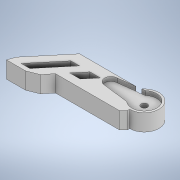
# Autodesk Inventor part: signle v2
Saved by Autodesk Inventor 2021 (Build 250183000, 183)
## iProperties
Created: 2022-04-17
Part Number: signle v2
Material: Genérico
Document SubType Name: Modeling
Designer: orgyn
Density: 1 g/cm^3
Appearance: Valor por defecto
Author: orgyn
Autodesk Inventor part; units mm, degrees
ref_plane "YZ Plane" through (0, 0, 0) normal (1, 0, 0) x (0, 1, 0)
ref_plane "XZ Plane" through (0, 0, 0) normal (0, 1, 0) x (-1, 0, 0)
ref_plane "XY Plane" through (0, 0, 0) normal (0, 0, 1) x (1, 0, 0)
sketch "Boceto1" plane through (0, 0, 0) normal (0, 1, 0) x (-1, 0, 0)
  line L0 (50, -16.5) -> (49.0807, -16.5)
  circle A0 centre (0, -33) radius 1.5
  circle A1 centre (0, -33) radius 3
  arc A2 (0, -26) -> (5.7446, -37) centre (0, -33) ccw
  line L1 (5.7446, -37) -> (35, -37)
  line L2 (35, -37) -> (50, -19)
  line L3 (0, -23) -> (20, -23)
  line L4 (20, -23) -> (20, -17)
  line L5 (20, -17) -> (50, -17)
  line L6 (50, -17) -> (50, -19)
  line L7 (0, -31.5) -> (0, -30)
  line L8 (0, -26) -> (0, -23)
  point P0 (0, -37)
  constraints: 18 end point, 3 coincident, 2 point on circle, 2 vertical alignment, 1 centre point, 1 vertical, 4 other
extrude "Extrusión1" add sketch "Boceto1" along normal blind 8 contours A1 | L8 L3 L4 L5 L6 L2 L1 A2
sketch "Boceto2" plane through (0, 8, 0) normal (0, 1, 0) x (1, 0, 0)
  circle A0 centre (0, 0) radius 3
  dimension "d12" = 6
  constraints: 1 centre point, 1 coincident
  measures "d12" diameter of A0
extrude "Extrusión2" cut sketch "Boceto2" against normal blind 4
sketch "Boceto6" plane through (0, 0, 0) normal (0, -1, 0) x (1, 0, 0)
  line L0 (-50, -17) -> (-20, -17) projected
  line L1 (-50, -16) -> (-50, -14) projected
  line L2 (-50, -17) -> (-50, -16)
  line L3 (-50, -16.5) -> (-16.403, -16.5)
  line L4 (-20, -23) -> (-25, -23)
  line L5 (-5.7446, -37) -> (-35, -37) projected
  line L6 (-25, -23) -> (-25, -28)
  line L7 (-25, -37) -> (-25, -32)
  line L8 (-25, -32) -> (-5.7446, -32)
  line L9 (-5.7446, -32) -> (-5.7446, -27.061)
  line L10 (-25, -28) -> (-5.7446, -28)
  line L11 (-35, -37) -> (-30, -37)
  line L12 (-30, -37) -> (-30, -32)
  line L13 (-30, -32) -> (-25, -32)
  line L14 (-50, -19) -> (-50, -17) projected
  line L15 (-50, -19) -> (-45, -19)
  line L16 (-30, -37) -> (-45, -19)
  line L17 (-45, -19) -> (-40, -19)
  line L18 (-30, -32) -> (-40.8333, -19)
  line L19 (-40.8333, -19) -> (-25, -19)
  line L20 (-25, -19) -> (-25, -28)
  line L21 (-30, -32) -> (-34.1667, -32)
  line L22 (-40.8333, -19) -> (-35.8333, -19)
  line L23 (-35.8333, -19) -> (-25, -32)
  line L24 (-35.8333, -19) -> (-30.8333, -19)
  line L25 (-25, -32) -> (-20, -32)
  line L26 (-20, -32) -> (-30.8333, -19)
  line L27 (-30, 4) -> (-45, -14)
  line L28 (-45, -14) -> (-40, -14)
  line L29 (-30, -1) -> (-40.8333, -14)
  line L30 (-30, -1) -> (-34.1667, -1)
  line L31 (-35.8333, -14) -> (-25, -1)
  line L32 (-35.8333, -14) -> (-30.8333, -14)
  line L33 (-25, -1) -> (-20, -1)
  line L34 (-20, -1) -> (-30.8333, -14)
  point P0 (0, 0)
  dimension "d28" = 5
  dimension "d29" = 5
  dimension "d30" = 5
  dimension "d31" = 5
  dimension "d32" = 5
  dimension "d33" = 5
  dimension "d34" = 5
  dimension "d35" = 5
  dimension "d36" = 5
  constraints: 62 end point, 12 point on line, 10 symmetric about line, 5 perpendicular, 3 horizontal, 3 parallel, 2 vertical, 1 collinear, 1 midpoint
  measures "d28" distance of L4.start L4.end
  measures "d29" distance of L4.end L6.end
  measures "d30" distance of L7.start L7.end
  measures "d31" distance of L5.end L11.end
  measures "d32" distance of L14.start L15.end
  measures "d33" distance of L15.end L17.end
  measures "d34" distance of L18.end L22.end
  measures "d35" distance of L22.end L24.end
  measures "d36" distance of L7.end L25.end
extrude "Extrusión6" cut sketch "Boceto6" against normal blind 10 contours L23 L19 L26 L6 L10 L8 | L21 L16 L17 L18 | L10 L6 L26 | L30 L29 L28 L27 | L31 L33 L34 L32
chamfer "Chaflán1" distance 2 angle 45 2 edges at (-50, 4, -19) (0, 4, -23)
sketch "Boceto9" plane through (0, 0, 0) normal (0, -1, 0) x (1, 0, 0)
  circle A0 centre (0, -33) radius 1.5 projected
  circle A1 centre (0, -33) radius 3
  point P0 (0, 0)
  dimension "d47" = 6
  constraints: 1 centre point, 1 coincident
  measures "d47" diameter of A1
extrude "Extrusión9" cut sketch "Boceto9" against normal blind 4
sketch "Boceto10" plane through (0, 8, 0) normal (0, 1, 0) x (1, 0, 0)
  circle A0 centre (0, 33) radius 1.5 projected
  circle A1 centre (0, 33) radius 6
  line L0 (0, 33) -> (-19, 33)
  line L1 (0, 33) -> (0, 37.5)
  line L2 (0, 37.5) -> (-19, 37.5)
  line L3 (-19, 37.5) -> (-19, 28.5)
  line L4 (-19, 28.5) -> (0, 28.5)
  line L5 (-19, 33) -> (-16, 33)
  circle A2 centre (-16, 33) radius 3
  circle A3 centre (-16, 33) radius 3
  line L6 (-16, 36) -> (-3.9686, 37.5)
  line L7 (-16, 33) -> (-16, 30)
  line L8 (-16, 30) -> (-3.9686, 28.5)
  point P0 (0, 0)
  dimension "d50" = 12
  dimension "d51" = 19
  dimension "d52" = 4.5
  dimension "d53" = 9
  dimension "d54" = 3
  constraints: 18 end point, 4 point on circle, 4 point on line, 3 coincident, 3 perpendicular, 2 centre point, 1 horizontal, 1 vertical, 4 other
  measures "d50" diameter of A1
  measures "d51" distance of L0.start L0.end
  measures "d52" distance of L0.start L1.end
  measures "d53" distance of L2.end L3.end
  measures "d54" distance of L0.end L5.end
extrude "Extrusión10" cut sketch "Boceto10" against normal blind 2 contours A0 L1 L2 A1 L0 | A0 L0 A1 L2 L1 | L0 A2 L6 A1 | A1 L8 A2 L0 | A2 L7 L0 | L0 A2 | A2 L0 L7
sketch "Boceto14" plane through (0, 0, 0) normal (0, -1, 0) x (1, 0, 0)
  line L0 (-40.8333, -14) -> (-30, -1) projected
  line L1 (-35.8333, -14) -> (-30.8333, -14) projected
  line L2 (-40.8333, -14) -> (-35.8333, -14)
  line L3 (-35.8333, -14) -> (-38.3333, -14)
  line L4 (-25, -1) -> (-35.8333, -14) projected
  line L5 (-35.8333, -14) -> (-29.4226, -6.3071)
  line L6 (-34.4226, -6.3071) -> (-29.4226, -6.3071)
  line L7 (-29.4226, -6.3071) -> (-20, -6.3071)
  line L8 (0, -10) -> (9, -10) projected
  line L9 (-20, -6.3071) -> (-20, -10)
  line L10 (-40.8333, -14) -> (-40.8333, -16)
  line L11 (-20, -16) -> (-50, -16) projected
  line L12 (-20, -10) -> (-20, -16) projected
  line L13 (-40.8333, -16) -> (-20, -16)
  line L14 (-20, -16) -> (-20, -10)
  line L15 (-35.8333, -14) -> (-30.8333, -14)
  line L16 (-30.8333, -14) -> (-20, -1) projected
  line L17 (-24.4226, -6.3071) -> (-30.8333, -14)
  line L18 (-35.8333, -14) -> (-40.8333, -16)
  line L19 (-50, -16) -> (-50, -17)
  line L20 (-50, -16.5) -> (-40.8333, -16.5)
  line L21 (-40.8333, -19) -> (-30, -32)
  line L22 (-35.8333, -19) -> (-30.8333, -19)
  line L23 (-40.8333, -19) -> (-35.8333, -19)
  line L24 (-35.8333, -19) -> (-38.3333, -19)
  line L25 (-25, -32) -> (-35.8333, -19)
  line L26 (-35.8333, -19) -> (-29.4226, -26.6929)
  line L27 (-34.4226, -26.6929) -> (-29.4226, -26.6929)
  line L28 (-29.4226, -26.6929) -> (-20, -26.6929)
  line L29 (-20, -26.6929) -> (-20, -23)
  line L30 (-40.8333, -19) -> (-40.8333, -17)
  line L31 (-20, -23) -> (-20, -17)
  line L32 (-40.8333, -17) -> (-20, -17)
  line L33 (-20, -17) -> (-20, -23)
  line L34 (-35.8333, -19) -> (-30.8333, -19)
  line L35 (-30.8333, -19) -> (-20, -32)
  line L36 (-24.4226, -26.6929) -> (-30.8333, -19)
  line L37 (-35.8333, -19) -> (-40.8333, -17)
  point P0 (0, 0)
  point P1 (7, -10)
  constraints: 62 end point, 15 point on line, 15 symmetric about line, 4 horizontal, 2 collinear, 2 midpoint, 1 perpendicular, 1 vertical
extrude "Extrusión13" cut sketch "Boceto14" against normal blind 8 contours L18 L1 L16 L7 L9 L12 L11 | L32 L31 L29 L28 L35 L22 L37
sketch "Boceto15" plane through (0, 0, 0) normal (0, -1, 0) x (1, 0, 0)
  line L0 (-20, -6.3071) -> (-24.4226, -6.3071) projected
  line L1 (-20, -6.3071) -> (-29.4226, -6.3071)
  line L2 (-35.8333, -14) -> (-25, -1) projected
  line L3 (-20, -10) -> (-20, -6.3071) projected
  line L4 (-20, -10) -> (-32.5381, -10)
  line L5 (-32.5381, -10) -> (-29.4226, -6.3071)
  line L6 (-50, -17) -> (-40.8333, -17) projected
  line L7 (-40.8333, -16) -> (-50, -16) projected
  line L8 (-50, -17) -> (-50, -16)
  line L9 (-50, -16.5) -> (-36.6527, -16.5)
  line L10 (-20, -26.6929) -> (-24.4226, -26.6929)
  line L11 (-20, -26.6929) -> (-29.4226, -26.6929)
  line L12 (-20, -23) -> (-20, -26.6929)
  line L13 (-20, -23) -> (-32.5381, -23)
  line L14 (-32.5381, -23) -> (-29.4226, -26.6929)
  point P0 (0, 0)
  point P1 (-32.5, -10)
  constraints: 20 end point, 5 symmetric about line, 3 horizontal, 1 midpoint, 1 point on line, 1 vertical
extrude "Extrusión14" add sketch "Boceto15" against normal blind 8 contours L3 L4 L2 L1 L0 | L10 L11 L14 L13 L12
sketch "Boceto17" plane through (0, 8, 0) normal (0, 1, 0) x (1, 0, 0)
  line L0 (-20, 10) -> (-32.5, 10) projected
  line L1 (-29.4226, 6.3071) -> (-20, 6.3071) projected
  line L2 (-32.5, 10) -> (-29.4226, 6.3071)
  line L3 (-29.4226, 6.3071) -> (-20, 6.3071)
  line L4 (-20, 6.3071) -> (-20, 10) projected
  line L5 (-20, 6.3071) -> (-20, 10)
  line L6 (-20, 10) -> (-32.5, 10)
  point P0 (0, 0)
  constraints: 8 end point, 2 collinear, 1 perpendicular
extrude "Extrusión16" cut sketch "Boceto17" against normal blind 10
